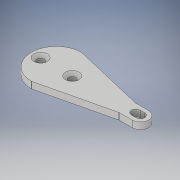
# Autodesk Inventor part: Деталь_1
Saved by Autodesk Inventor 2019 (Build 230136000, 136)
## iProperties
Created: 2020-04-06
Part Number: Деталь_1
Material: Типовые
Document SubType Name: Modeling
Designer: Diana
Density: 1 g/cm^3
Appearance: По умолчанию
Author: Diana
Autodesk Inventor part; units mm, degrees
ref_plane "YZ Plane" through (0, 0, 0) normal (1, 0, 0) x (0, 1, 0)
ref_plane "XZ Plane" through (0, 0, 0) normal (0, 1, 0) x (-1, 0, 0)
ref_plane "XY Plane" through (0, 0, 0) normal (0, 0, 1) x (1, 0, 0)
sketch "Эскиз1" plane through (0, 0, 0) normal (0, 1, 0) x (-1, 0, 0)
  arc A0 (0, -38) -> (0, 38) centre (0, 0) ccw
  line L0 (0, 38) -> (-107.5, 12.5)
  line L1 (0, -38) -> (-107.5, -12.5)
  line L2 (0, -53.2) -> (0, 53.2) projected
  line L3 (-107.5, 12.5) -> (-127.5, 12.5)
  line L4 (-107.5, -12.5) -> (-127.5, -12.5)
  arc A1 (-127.5, 12.5) -> (-127.5, -12.5) centre (-127.5, 0) ccw
  line L5 (-120.5, 6.5) -> (-127.5, 6.5)
  line L6 (-120.5, -6.5) -> (-127.5, -6.5)
  arc A2 (-120.5, -6.5) -> (-120.5, 6.5) centre (-120.5, 0) ccw
  arc A3 (-127.5, 6.5) -> (-127.5, -6.5) centre (-127.5, 0) ccw
  point P0 (-117.5, 12.5)
  dimension "d0" = 38
  dimension "d7" = 20
  dimension "d8" = 25
  dimension "d9" = 127.5
  dimension "d10" = 12.5
  dimension "d11" = 13
  dimension "d12" = 7
  constraints: 12 end point, 8 point on circle, 5 vertical alignment, 4 centre point, 4 horizontal, 3 equal length, 3 point on line, 2 coincident, 1 midpoint, 1 tangent, 1 other
  measures "d0" radius of A0
  measures "d7" distance of L0.end L3.end
  measures "d8" distance between parallel lines of L4 L3
  measures "d9" distance of point (0, 0) A1.centre
  measures "d10" radius of A1
  measures "d11" distance between parallel lines of L6 L5
  measures "d12" distance of A3.centre A2.centre
extrude "Выдавливание1" add sketch "Эскиз1" along normal blind 10
sketch "Эскиз2" plane through (0, 10, 0) normal (0, 1, 0) x (1, 0, 0)
  point P0 (0, 0)
  point P1 (-24, 0)
  point P2 (24, 0)
  dimension "d15" = 24
  dimension "d16" = 48
  constraints: 2 horizontal alignment
  measures "d15" distance of point (-24, 0) point (0, 0)
  measures "d16" distance of point (24, 0) point (-24, 0)
hole "Отверстие1" at (-24, 10, 0) at (24, 10, 0) direction (0, -1, 0) diameter 11 end through all countersink diameter 20.4 countersink angle 90 clearance for "Винт крепежный с полупотайной головкой" size "M10" standard "ANSI метрическая"
fillet "Сопряжение1" radius 2 4 edges at (0, 5, 38) (0, 5, -38) (107.5, 5, -12.5) (107.5, 5, 12.5)
